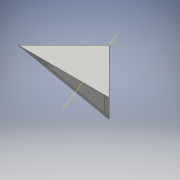
# Autodesk Inventor part: Part2-01
Saved by Autodesk Inventor 2016 (Build 200138000, 138)
## iProperties
Created: 2016-06-30
Part Number: Part2-01
Material: Generic
Document SubType Name: Modeling
Designer: kam42
Density: 1 g/cm^3
Appearance: Default
Author: kam42
Autodesk Inventor part; units mm, degrees
ref_plane "YZ Plane" through (0, 0, 0) normal (1, 0, 0) x (0, 1, 0)
ref_plane "XZ Plane" through (0, 0, 0) normal (0, 1, 0) x (-1, 0, 0)
ref_plane "XY Plane" through (0, 0, 0) normal (0, 0, 1) x (1, 0, 0)
sketch "Sketch3" plane through (0, 0, 0) normal (0, 0, 1) x (1, 0, 0)
  line L0 (0, 27.3333) -> (-41, -13.6667)
  line L1 (-41, -13.6667) -> (41, -13.6667)
  line L2 (41, -13.6667) -> (0, 27.3333)
  line L3 (41, -13.6667) -> (-20.5, 6.8333) construction
  line L4 (-41, -13.6667) -> (20.5, 6.8333) construction
  point P0 (0, 0)
  dimension "d7" = 90
  dimension "d8" = 45
  dimension "d9" = 82
  constraints: 10 end point, 2 midpoint, 2 point on line, 1 horizontal
  measures "d7" angle of L2 L0
  measures "d8" angle of L1 L0
  measures "d9" distance of L0.end L1.end
extrude "Extrusion1" add sketch "Sketch3" against normal blind 3 draft -45
sketch "Sketch4" plane through (0, 0, 0) normal (0, 0, 1) x (1, 0, 0)
  line L0 (-33.7574, -10.6667) -> (33.7574, -10.6667) projected
  line L1 (0, 23.0907) -> (-33.7574, -10.6667) projected
  point P0 (0, 0)
  point P1 (0, -10.6667)
  constraints: 1 midpoint
ref_plane "Work Plane2" through (0, -10.6667, 0) normal (-1, 0, 0) x (0, 1, 0)
sketch "Sketch5" plane through (0, -10.6667, 0) normal (-1, 0, 0) x (0, 1, 0)
  line L0 (38, 0) -> (-3, 0) construction
  line L1 (-3, 0) -> (10.6667, 19.3276) construction
  line L2 (38, 0) -> (10.6667, 19.3276)
  line L3 (-3, 0) -> (38, 0) projected
  point P0 (10.6667, 0)
  dimension "d18" = 23.6714
  constraints: 4 end point, 1 perpendicular
  measures "d18" distance of L0.end L1.end
pattern_circular "Circular Pattern1" count 3 over 360 about axis through (0, 27.3333, 0) along (0, -0.8164966, -0.5773503) of "Extrusion1"
sketch "Sketch6" plane through (0, -10.6667, 0) normal (-1, 0, 0) x (0, 1, 0)
  line L0 (38, 0) -> (-3, 0) projected
  line L1 (38, 0) -> (38, 57.9828) projected
  line L2 (38, 57.9828) -> (-3, 0) projected
  line L3 (38, 0) -> (-3, 0) projected
  line L4 (48.9333, -7.731) -> (-27.6, 46.3862) projected
  point P0 (10.6667, 0)
  point P1 (25.7526, 8.6603)
  dimension "d20" = 15
  constraints: 1 point on line
  measures "d20" distance of point (25.753, 8.66) L0.start
ref_plane "Work Plane4" through (0, 15.0859, -8.6603) normal (0, 0.8164966, 0.5773503) x (1, 0, 0)
ref_plane "Work Plane3" through (-41, -13.6667, 0) normal (0, 0.8164966, 0.5773503) x (1, 0, 0)
sketch "Sketch7" plane through (0, 15.0859, -8.6603) normal (0, 0.8164966, 0.5773503) x (1, 0, 0)
  line L0 (12.0072, -6.9324) -> (0, 13.8647) projected
  line L1 (0, 13.8647) -> (-12.0072, -6.9324) projected
  line L2 (-12.0072, -6.9324) -> (12.0072, -6.9324) projected
  line L3 (0, 21.2132) -> (18.3712, -10.6066) projected
  line L4 (18.3712, -10.6066) -> (-18.3712, -10.6066) projected
  line L5 (-18.3712, -10.6066) -> (0, 21.2132) projected
  line L6 (-12.0072, -6.9324) -> (0, 13.8647)
  line L7 (12.0072, -6.9324) -> (0, 13.8647)
  line L8 (12.0072, -6.9324) -> (-12.0072, -6.9324)
  point P0 (0, -15.7809)
  constraints: 6 end point, 2 collinear
extrude "Extrusion2" add sketch "Sketch7" along normal up to next contours L2 L1 L0
body "Solid1"
